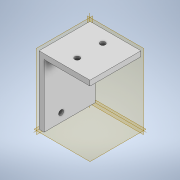
# Autodesk Inventor part: T_shape
Saved by Autodesk Inventor 2022 (Build 260153000, 153)
## iProperties
Created: 2022-05-11
Part Number: T_shape
Material: Generic
Document SubType Name: Modeling
Designer: dovalle
Density: 1 g/cm^3
Appearance: Default
Author: dovalle
Autodesk Inventor part; units mm, degrees
sketch "Sketch1" plane through (0, 0, 0) normal (0, 0, 1) x (1, 0, 0)
  line L0 (0, 0) -> (0, 40)
  line L1 (0, 40) -> (30, 40)
  line L2 (30, 40) -> (30, 37)
  line L3 (30, 37) -> (3, 37)
  line L4 (3, 37) -> (3, 0)
  line L5 (3, 0) -> (0, 0)
  constraints: 12 end point, 4 perpendicular, 1 parallel, 1 vertical
extrude "Extrusion1" add sketch "Sketch1" along normal blind 30
sketch "Sketch2" plane through (3, 0, 0) normal (1, 0, 0) x (0, 0, -1)
  line L0 (-30, 37) -> (-30, 40) projected
  line L1 (-30, 40) -> (-20, 40)
  line L2 (0, 40) -> (-30, 40) projected
  line L3 (0, 0) -> (-30, 0) projected
  line L4 (-20, 0) -> (-10, 0)
  line L5 (0, 37) -> (-30, 37) projected
  circle A0 centre (-20, 32) radius 1.5
  circle A1 centre (-20, 5) radius 1.5
  circle A2 centre (-10, 20) radius 1.5
  constraints: 4 end point, 3 centre point, 3 point on line
extrude "Extrusion2" cut sketch "Sketch2" against normal blind 30
sketch "Sketch3" plane through (0, 40, 0) normal (0, 1, 0) x (1, 0, 0)
  line L0 (0, 0) -> (0, -30) projected
  line L1 (3, 0) -> (30, 0) projected
  line L2 (3, -30) -> (30, -30) projected
  circle A0 centre (15, -15) radius 1.5
  constraints: 1 centre point
extrude "Extrusion3" cut sketch "Sketch3" against normal blind 30
sketch "Sketch4" plane through (0, 40, 0) normal (0, 1, 0) x (1, 0, 0)
  circle A0 centre (15, -15) radius 1.5 projected
  circle A1 centre (15, -15) radius 1.5
  point P0 (0, 0)
  constraints: 1 centre point, 1 coincident
extrude "Extrusion4" add sketch "Sketch4" against normal blind 3
sketch "Sketch5" plane through (0, 40, 0) normal (0, 1, 0) x (1, 0, 0)
  point P0 (0, 0)
sketch "Sketch6" plane through (0, 40, 0) normal (0, 1, 0) x (1, 0, 0)
  line L0 (3, -30) -> (30, -30) projected
  circle A0 centre (15, -22.5) radius 1.5
  circle A1 centre (15, -7.5) radius 1.5
  point P0 (0, 0)
  constraints: 2 centre point
extrude "Extrusion5" cut sketch "Sketch6" against normal blind 3
body "Solid1"
